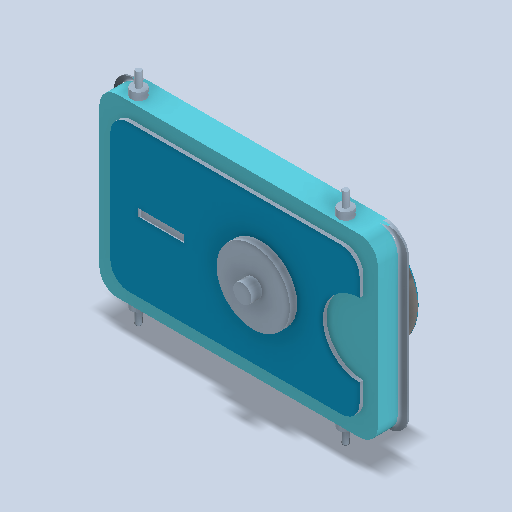
# Autodesk Inventor part: project_part
Saved by Autodesk Inventor 2024 (Build 280153000, 153)
## iProperties
Created: 2023-06-10
Part Number: project_part
Material: Generic
Document SubType Name: Modeling
Designer: gaura
Density: 1 g/cm^3
Appearance: Steel Blue
Author: gaura
Autodesk Inventor part; units mm, degrees
ref_plane "YZ Plane" through (0, 0, 0) normal (1, 0, 0) x (0, 1, 0)
ref_plane "XZ Plane" through (0, 0, 0) normal (0, 1, 0) x (-1, 0, 0)
ref_plane "XY Plane" through (0, 0, 0) normal (0, 0, 1) x (1, 0, 0)
sketch "Sketch1" plane through (0, 0, 0) normal (0, 0, 1) x (1, 0, 0)
  line L0 (-190, -120) -> (190, -120)
  line L1 (190, -120) -> (190, 120)
  line L2 (190, 120) -> (-190, 120)
  line L3 (-190, 120) -> (-190, -120)
  line L4 (-190, -120) -> (190, 120) construction
  line L5 (190, -120) -> (-190, 120) construction
  point P0 (0, 0)
  dimension "d0" = 380
  dimension "d1" = 240
  constraints: 12 end point, 2 midpoint, 2 parallel, 1 horizontal, 1 perpendicular
  measures "d0" distance of L2.end L1.end
  measures "d1" distance of L1.end L0.end
extrude "Extrusion1" add sketch "Sketch1" along normal blind 30
sketch "Sketch2" plane through (0, 0, 30) normal (0, 0, 1) x (1, 0, 0)
  line L0 (-170, -100) -> (170, -100)
  line L1 (170, -100) -> (170, 100)
  line L2 (170, 100) -> (-170, 100)
  line L3 (-170, 100) -> (-170, -100)
  line L4 (-170, -100) -> (170, 100) construction
  line L5 (170, -100) -> (-170, 100) construction
  point P0 (0, 0)
  dimension "d4" = 340
  dimension "d5" = 200
  constraints: 12 end point, 2 midpoint, 2 parallel, 1 horizontal, 1 perpendicular
  measures "d4" distance of L2.end L1.end
  measures "d5" distance of L1.end L0.end
extrude "Extrusion2" add sketch "Sketch2" along normal blind 5
fillet "Fillet1" radius 25 8 edges at (-190, 120, 15) (-170, 100, 32.5) (190, 120, 15) (170, 100, 32.5) (190, -120, 15) (170, -100, 32.5) (-170, -100, 32.5) (-190, -120, 15)
sketch "Sketch3" plane through (0, 0, 35) normal (0, 0, 1) x (1, 0, 0)
  line L0 (170, 75) -> (170, -75) projected
  arc A0 (170, 75) -> (145, 100) centre (145, 75) ccw projected
  arc A1 (170, 50) -> (170, -50) centre (170, 0) ccw
  point P0 (0, 0)
  dimension "d41" = 100
  constraints: 2 point on circle, 2 point on line, 1 centre point, 1 midpoint
  measures "d41" diameter of A1
extrude "Extrusion3" cut sketch "Sketch3" against normal blind 5
sketch "Sketch4" plane through (0, 0, 35) normal (0, 0, 1) x (1, 0, 0)
  circle A0 centre (35, 0) radius 50
  line L0 (-190, 95) -> (-190, -95) projected
  point P0 (0, 0)
  dimension "d48" = 100
  dimension "d49" = 225
  constraints: 1 centre point
  measures "d48" diameter of A0
  measures "d49" distance from line of A0.centre L0
extrude "Extrusion4" add sketch "Sketch4" along normal blind 10
sketch "Sketch6" plane through (0, 0, 0) normal (0, 0, -1) x (-1, 0, 0)
  line L0 (200, 120) -> (-200, 120)
  line L1 (-200, 120) -> (-200, -120)
  line L2 (-200, -120) -> (200, -120)
  line L3 (200, -120) -> (200, 120)
  line L4 (200, 120) -> (-200, -120) construction
  line L5 (-200, 120) -> (200, -120) construction
  point P0 (0, 0)
  dimension "d18" = 400
  dimension "d19" = 240
  constraints: 12 end point, 2 midpoint, 2 parallel, 1 horizontal, 1 perpendicular
  measures "d18" distance of L2.end L1.end
  measures "d19" distance of L1.end L0.end
extrude "Extrusion6" add sketch "Sketch6" along normal blind 2.5
fillet "Fillet3" radius 3 6 edges at (-190, 0, 0) (-182.6777, 112.6777, 0) (-182.6777, -112.6777, 0) (190, 0, 0) (182.6777, 112.6777, 0) (182.6777, -112.6777, 0)
fillet "Fillet4" radius 25 4 edges at (200, 120, -1.25) (200, -120, -1.25) (-200, 120, -1.25) (-200, -120, -1.25)
sketch "Sketch7" plane through (0, 0, -2.5) normal (0, 0, -1) x (-1, 0, 0)
  line L0 (-190, -120) -> (190, -120)
  line L1 (190, -120) -> (190, 120)
  line L2 (190, 120) -> (-190, 120)
  line L3 (-190, 120) -> (-190, -120)
  line L4 (-190, -120) -> (190, 120) construction
  line L5 (190, -120) -> (-190, 120) construction
  point P0 (0, 0)
  dimension "d24" = 380
  dimension "d25" = 240
  constraints: 12 end point, 2 midpoint, 2 parallel, 1 horizontal, 1 perpendicular
  measures "d24" distance of L2.end L1.end
  measures "d25" distance of L1.end L0.end
extrude "Extrusion7" add sketch "Sketch7" along normal blind 5
fillet "Fillet5" radius 25 4 edges at (190, 120, -5) (-190, 120, -5) (-190, -120, -5) (190, -120, -5)
sketch "Sketch8" plane through (0, 0, -7.5) normal (0, 0, -1) x (-1, 0, 0)
  circle A0 centre (0, 0) radius 8.7919 projected
  circle A1 centre (-95, 0) radius 75
  circle A2 centre (95, 0) radius 75
  dimension "d30" = 150
  dimension "d32" = 150
  dimension "d44" = 95
  dimension "d45" = 95
  constraints: 2 centre point
  measures "d30" diameter of A1
  measures "d32" diameter of A2
  measures "d44" distance of A1.centre point (0, 0)
  measures "d45" distance of A2.centre point (0, 0)
extrude "Extrusion8" add sketch "Sketch8" along normal blind 40 contours A1 | A2
fillet "Fillet6" radius 3 2 edges at (170, 0, -47.5) (-20, 0, -47.5)
sketch "Sketch9" plane through (0, 0, 35) normal (0, 0, 1) x (1, 0, 0)
  arc A0 (-165, 120) -> (-190, 95) centre (-165, 95) ccw projected
  line L0 (-130, -5) -> (-70, -5)
  line L1 (-70, -5) -> (-70, 5)
  line L2 (-70, 5) -> (-130, 5)
  line L3 (-130, 5) -> (-130, -5)
  line L4 (-130, -5) -> (-70, 5) construction
  line L5 (-70, -5) -> (-130, 5) construction
  point P0 (0, 0)
  point P1 (-100, 0)
  point P2 (-100, 0)
  point P3 (-100, 0)
  dimension "d36" = 60
  dimension "d37" = 10
  dimension "d42" = 0
  dimension "d43" = 100
  constraints: 12 end point, 4 midpoint, 2 parallel, 1 horizontal, 1 perpendicular
  measures "d36" distance of L2.end L1.end
  measures "d37" distance of L1.end L0.end
  measures "d42" vertical distance of point (0, 0) point (-100, 0)
  measures "d43" distance of point (-100, 0) point (0, 0)
extrude "Extrusion9" cut sketch "Sketch9" against normal blind 1.5
fillet "Fillet7" radius 2 1 edges at (-130, 0, 35)
sketch "Sketch10" plane through (35, 0, 45) normal (0, 0, 1) x (1, 0, 0)
  circle A0 centre (0, 0) radius 12.5
  circle A1 centre (0, 0) radius 50 projected
  point P0 (-35, 0)
  dimension "d50" = 25
  constraints: 1 centre point, 1 concentric
  measures "d50" diameter of A0
extrude "Extrusion10" add sketch "Sketch10" along normal blind 15 contours A0
sketch "Sketch11" plane through (0, 0, 0) normal (0, 1, 0) x (-1, 0, 0)
  line L0 (-190, 3) -> (-190, 30) construction
  line L1 (-190, 16.5) -> (190, 16.5) construction
  line L2 (190, 30) -> (190, 3) construction
  circle A0 centre (-132.5, 16.5) radius 10
  circle A1 centre (150, 16.5) radius 10
  point P0 (0, 0)
  dimension "d53" = 20
  dimension "d54" = 20
  dimension "d55" = 57.5
  dimension "d56" = 40
  constraints: 2 centre point, 2 end point, 2 midpoint, 2 point on line
  measures "d53" diameter of A0
  measures "d54" diameter of A1
  measures "d55" distance from line of A0.centre L0
  measures "d56" distance from line of L2 A1.centre
extrude "Extrusion11" add sketch "Sketch11" along normal mid plane 260
sketch "Sketch12" plane through (0, 0, 0) normal (0, 1, 0) x (-1, 0, 0)
  line L0 (-190, 3) -> (-190, 30) construction
  line L1 (-190, 16.5) -> (190, 16.5) construction
  line L2 (190, 30) -> (190, 3) construction
  circle A0 centre (-132.5, 16.5) radius 4
  circle A1 centre (150, 16.5) radius 4
  point P0 (0, 0)
  dimension "d59" = 8
  dimension "d60" = 8
  constraints: 2 centre point, 2 coincident, 2 end point, 2 midpoint
  measures "d59" diameter of A0
  measures "d60" diameter of A1
extrude "Extrusion12" add sketch "Sketch12" along normal mid plane 300
body "Solid1"
